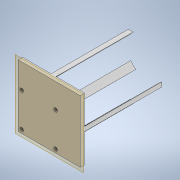
# Autodesk Inventor part: nema34
Saved by Autodesk Inventor 2020 (Build 240168000, 168)
## iProperties
Created: 2021-09-05
Part Number: nema34
Material: Generic
Document SubType Name: Modeling
Designer: super
Density: 1 g/cm^3
Appearance: Default
Author: super
Autodesk Inventor part; units mm, degrees
ref_plane "YZ Plane" through (0, 0, 0) normal (1, 0, 0) x (0, 1, 0)
ref_plane "XZ Plane" through (0, 0, 0) normal (0, 1, 0) x (-1, 0, 0)
sketch "Sketch1" plane through (0, 0, 0) normal (0, 0, 1) x (1, 0, 0)
  line L0 (0, 0) -> (86, 0)
  line L1 (86, 0) -> (86, 86)
  line L2 (86, 86) -> (0, 86)
  line L3 (0, 86) -> (0, 0)
  circle A0 centre (5, 5) radius 2.5
  circle A1 centre (52, 5) radius 2.5
  circle A2 centre (5, 52) radius 2.5
  circle A3 centre (52, 52) radius 2.5
  dimension "d0" = 86
  dimension "d1" = 86
  dimension "d2" = 5
  dimension "d3" = 5
  dimension "d4" = 5
  constraints: 8 end point, 4 centre point, 2 parallel, 1 horizontal, 1 perpendicular
  measures "d0" distance of L2.end L1.end
  measures "d1" distance of L1.end L0.end
  measures "d2" diameter of A0
  measures "d3" horizontal distance of L0.start A0.centre
  measures "d4" horizontal distance of L0.start A0.centre
extrude "Extrusion1" add sketch "Sketch1" against normal blind 113
sketch "Sketch2" plane through (0, 0, -113) normal (0, 0, -1) x (-1, 0, 0)
  line L0 (0, 86) -> (-86, 86) projected
  line L1 (-43, 86) -> (-43, 0)
  line L2 (-86, 0) -> (0, 0) projected
  line L3 (-86, 86) -> (-86, 0) projected
  line L4 (-86, 43) -> (0, 43)
  line L5 (0, 0) -> (0, 86) projected
  arc A0 (-46.3441, 0) -> (-86, 39.9524) centre (-66.1721, 19.9762) ccw
  line L6 (-86, 39.9524) -> (-86, 0)
  line L7 (0, 0) -> (-86, 0)
  line L8 (0, 86) -> (0, 0)
  arc A1 (0, 39.9524) -> (-39.6559, 0) centre (-19.8279, 19.9762) ccw
  line L9 (-86, 86) -> (0, 86)
  arc A2 (-86, 46.0476) -> (-46.3441, 86) centre (-66.1721, 66.0238) ccw
  line L10 (-86, 46.0476) -> (-86, 86)
  arc A3 (-39.6559, 86) -> (0, 46.0476) centre (-19.8279, 66.0238) ccw
  line L11 (0, 86) -> (-86, 86)
  point P0 (0, 39.9524)
  point P1 (-39.6559, 0)
  point P2 (-39.6559, 86)
  point P3 (0, 46.0476)
  point P4 (-86, 46.0476)
  point P5 (-46.3441, 86)
  constraints: 16 end point, 15 symmetric about line, 8 point on circle, 6 point on line, 4 centre point, 4 midpoint, 1 vertical, 3 other
extrude "Extrusion2" cut sketch "Sketch2" against normal blind 107 contours L5 A3 A1 A2 L0 | A2 L1 | A3 A2 A0 L3 L0 | L1 A3 | A3 L4 | L4 A1 | A1 L5 L2 A0 A3 | A2 L4 | L4 A0 | A0 A1 L2 L3 A2 | A0 L1 | L1 A1
body "Solid1"
